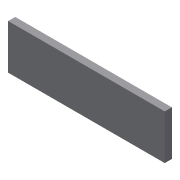
# Autodesk Inventor part: Zapata_freno
Saved by Autodesk Inventor 2020 (Build 240168000, 168)
## iProperties
Created: 2020-03-11
Part Number: Zapata_freno
Material: Generic
Document SubType Name: Modeling
Designer: Juan Carlos Botero
Density: 1 g/cm^3
Appearance: Default
Author: Juan Carlos Botero
Autodesk Inventor part; units mm, degrees
ref_plane "YZ Plane" through (0, 0, 0) normal (1, 0, 0) x (0, 1, 0)
ref_plane "XZ Plane" through (0, 0, 0) normal (0, 1, 0) x (-1, 0, 0)
ref_plane "XY Plane" through (0, 0, 0) normal (0, 0, 1) x (1, 0, 0)
sketch "Sketch1" plane through (0, 0, 0) normal (0, 0, 1) x (1, 0, 0)
  line L0 (-70, -20) -> (70, -20)
  line L1 (70, -20) -> (70, 20)
  line L2 (70, 20) -> (-70, 20)
  line L3 (-70, 20) -> (-70, -20)
  line L4 (-70, -20) -> (70, 20) construction
  line L5 (70, -20) -> (-70, 20) construction
  point P0 (0, 0)
  dimension "d0" = 140
  dimension "d1" = 40
  constraints: 12 end point, 2 midpoint, 2 parallel, 1 horizontal, 1 perpendicular
  measures "d0" distance of L2.end L1.end
  measures "d1" distance of L1.end L0.end
extrude "Extrusion1" add sketch "Sketch1" along normal blind 6.35
sketch "Sketch2" plane through (0, 0, 0) normal (0, 0, -1) x (-1, 0, 0)
  circle A0 centre (-50, 0) radius 4
  circle A1 centre (0, 10) radius 4
  circle A2 centre (50, 0) radius 4
  line L0 (-70, -20) -> (-70, 20) projected
  point P0 (0, 0)
  point P1 (-70, 0)
  dimension "d4" = 20
  dimension "d5" = 100
  dimension "d6" = 50
  dimension "d7" = 8
  dimension "d8" = 10
  constraints: 3 centre point, 2 equal radius, 2 horizontal alignment, 1 midpoint
  measures "d4" distance from line of L0 A0.centre
  measures "d5" distance of A2.centre A0.centre
  measures "d6" horizontal distance of A0.centre A1.centre
  measures "d7" diameter of A1
  measures "d8" vertical distance of A0.centre A1.centre
extrude "Extrusion2" cut sketch "Sketch2" against normal through all
thicken "Thicken1" operation add thickness 5 both sides no extend neighbours yes toward (0, 1, 0) faces at (23.3333, 20, 2.1167)
body "Solid1"
